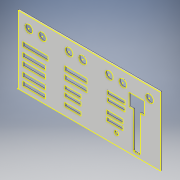
# Autodesk Inventor part: CNC - Tool Board
Saved by Autodesk Inventor 2017 SP1 (Build 210196100, 196)
## iProperties
Created: 2017-08-31
Part Number: CNC - Tool Board
Material: Generic
Document SubType Name: Modeling
Designer: rmainhar
Density: 1 g/cm^3
Appearance: Default
Author: rmainhar
Autodesk Inventor part; units mm, degrees
ref_plane "YZ Plane" through (0, 0, 0) normal (1, 0, 0) x (0, 1, 0)
ref_plane "XZ Plane" through (0, 0, 0) normal (0, 1, 0) x (-1, 0, 0)
ref_plane "XY Plane" through (0, 0, 0) normal (0, 0, 1) x (1, 0, 0)
sketch "Sketch1" plane through (0, 0, 0) normal (0, 0, 1) x (1, 0, 0)
  line L0 (0, 0) -> (584.2, 0)
  line L1 (584.2, 0) -> (584.2, 279.4)
  line L2 (584.2, 279.4) -> (0, 279.4)
  line L3 (0, 279.4) -> (0, 0)
  dimension "d0" = 584.2
  dimension "d1" = 279.4
  constraints: 8 end point, 2 parallel, 1 horizontal, 1 perpendicular
  measures "d0" distance of L2.end L1.end
  measures "d1" distance of L1.end L0.end
extrude "Extrusion1" add sketch "Sketch1" along normal blind 6.35
sketch "Sketch2" plane through (0, 0, 6.35) normal (0, 0, 1) x (1, 0, 0)
  circle A0 centre (43.6149, 234.95) radius 15.875
  circle A1 centre (99.4949, 234.95) radius 15.875
  line L0 (584.2, 279.4) -> (0, 279.4) projected
  circle A2 centre (208.7149, 234.95) radius 15.875
  circle A3 centre (264.5949, 234.95) radius 15.875
  circle A4 centre (373.8149, 234.95) radius 15.875
  circle A5 centre (429.6949, 234.95) radius 15.875
  circle A6 centre (538.9149, 234.95) radius 15.875
  circle A7 centre (594.7949, 234.95) radius 15.875
  point P0 (0, 0)
  dimension "d4" = 31.75
  dimension "d5" = 31.75
  dimension "d6" = 55.88
  dimension "d7" = 44.45
  dimension "d8" = 44.45
  dimension "d11" = 165.1
  constraints: 8 centre point, 1 horizontal, 12 other
  measures "d4" diameter of A0
  measures "d5" diameter of A1
  measures "d6" distance of A1.centre A0.centre
  measures "d7" distance from line of A1.centre L0
  measures "d8" distance from line of L0 A0.centre
  measures "d11" distance of A0.centre A2.centre
extrude "Extrusion2" cut sketch "Sketch2" against normal through all contours A0 | A1 | A2 | A3 | A4 | A5 | A6
sketch "Sketch3" plane through (0, 0, 6.35) normal (0, 0, 1) x (1, 0, 0)
  circle A0 centre (429.6949, 234.95) radius 15.875 projected
  circle A1 centre (264.5949, 234.95) radius 15.875 projected
  circle A2 centre (99.4949, 234.95) radius 15.875 projected
  circle A3 centre (43.6149, 234.95) radius 15.875 projected
  circle A4 centre (208.7149, 234.95) radius 15.875 projected
  circle A5 centre (373.8149, 234.95) radius 15.875 projected
  circle A6 centre (538.9149, 234.95) radius 15.875 projected
  line L0 (0, 0) -> (584.2, 0) projected
  line L1 (584.2, 0) -> (584.2, 279.4) projected
  line L2 (584.2, 279.4) -> (0, 279.4) projected
  line L3 (0, 279.4) -> (0, 0) projected
  line L4 (19.05, 177.8) -> (121.92, 177.8)
  line L5 (121.92, 177.8) -> (121.92, 158.75)
  line L6 (121.92, 158.75) -> (19.05, 158.75)
  line L7 (19.05, 158.75) -> (19.05, 177.8)
  line L8 (19.05, 139.7) -> (111.125, 139.7)
  line L9 (111.125, 139.7) -> (111.125, 120.65)
  line L10 (111.125, 120.65) -> (19.05, 120.65)
  line L11 (19.05, 120.65) -> (19.05, 139.7)
  line L12 (111.125, 107.95) -> (111.125, 88.9)
  line L13 (19.05, 107.95) -> (111.125, 107.95)
  line L14 (111.125, 88.9) -> (19.05, 88.9)
  line L15 (19.05, 88.9) -> (19.05, 107.95)
  line L16 (19.05, 50.8) -> (19.05, 69.85)
  line L17 (19.05, 19.05) -> (19.05, 38.1)
  line L18 (19.05, 69.85) -> (111.125, 69.85)
  line L19 (111.125, 69.85) -> (111.125, 50.8)
  line L20 (111.125, 50.8) -> (19.05, 50.8)
  line L21 (19.05, 38.1) -> (111.125, 38.1)
  line L22 (111.125, 38.1) -> (111.125, 19.05)
  line L23 (111.125, 19.05) -> (19.05, 19.05)
  dimension "d18" = 101.6
  dimension "d19" = 19.05
  dimension "d20" = 102.87
  dimension "d21" = 19.05
  dimension "d22" = 19.05
  dimension "d23" = 92.075
  dimension "d24" = 19.05
  dimension "d25" = 92.075
  dimension "d26" = 19.05
  dimension "d27" = 19.05
  dimension "d28" = 139.7
  dimension "d29" = 171.45
  dimension "d32" = 69.85
  constraints: 40 end point, 6 parallel, 3 horizontal, 3 perpendicular, 1 vertical, 16 other
  measures "d18" distance between parallel lines of L2 L4
  measures "d19" distance of L4.end L5.end
  measures "d20" distance between parallel lines of L5 L7
  measures "d21" distance between parallel lines of L3 L7
  measures "d22" distance of L9.start L9.end
  measures "d23" distance between parallel lines of L9 L11
  measures "d24" distance of L12.start L12.end
  measures "d25" distance between parallel lines of L12 L15
  measures "d26" distance between parallel lines of L3 L11
  measures "d27" distance between parallel lines of L15 L3
  measures "d28" distance between parallel lines of L2 L8
  measures "d29" distance between parallel lines of L2 L13
  measures "d32" distance of L8.start L16.end
extrude "Extrusion3" cut sketch "Sketch3" against normal through all contours L4 L5 L6 L7 | L8 L9 L10 L11 | L12 L14 L15 L13 | L16 L18 L19 L20 | L17 L21 L22 L23
sketch "Sketch4" plane through (0, 0, 6.35) normal (0, 0, 1) x (1, 0, 0)
  line L0 (19.05, 19.05) -> (19.05, 38.1) projected
  line L1 (19.05, 38.1) -> (111.125, 38.1) projected
  line L2 (111.125, 38.1) -> (111.125, 19.05) projected
  line L3 (111.125, 19.05) -> (19.05, 19.05) projected
  line L4 (19.05, 88.9) -> (19.05, 107.95) projected
  line L5 (19.05, 107.95) -> (111.125, 107.95) projected
  line L6 (111.125, 107.95) -> (111.125, 88.9) projected
  line L7 (111.125, 88.9) -> (19.05, 88.9) projected
  line L8 (19.05, 120.65) -> (19.05, 139.7) projected
  line L9 (19.05, 139.7) -> (111.125, 139.7) projected
  line L10 (111.125, 139.7) -> (111.125, 120.65) projected
  line L11 (111.125, 120.65) -> (19.05, 120.65) projected
  line L12 (19.05, 50.8) -> (19.05, 69.85) projected
  line L13 (19.05, 69.85) -> (111.125, 69.85) projected
  line L14 (111.125, 69.85) -> (111.125, 50.8) projected
  line L15 (111.125, 50.8) -> (19.05, 50.8) projected
  line L16 (19.05, 158.75) -> (19.05, 177.8) projected
  line L17 (19.05, 177.8) -> (121.92, 177.8) projected
  line L18 (121.92, 177.8) -> (121.92, 158.75) projected
  line L19 (121.92, 158.75) -> (19.05, 158.75) projected
  circle A0 centre (429.6949, 234.95) radius 15.875 projected
  circle A1 centre (264.5949, 234.95) radius 15.875 projected
  circle A2 centre (99.4949, 234.95) radius 15.875 projected
  circle A3 centre (43.6149, 234.95) radius 15.875 projected
  circle A4 centre (208.7149, 234.95) radius 15.875 projected
  circle A5 centre (373.8149, 234.95) radius 15.875 projected
  circle A6 centre (538.9149, 234.95) radius 15.875 projected
  line L20 (0, 0) -> (584.2, 0) projected
  line L21 (584.2, 0) -> (584.2, 279.4) projected
  line L22 (584.2, 279.4) -> (0, 279.4) projected
  line L23 (0, 279.4) -> (0, 0) projected
  line L24 (190.5, 158.75) -> (190.5, 177.8)
  line L25 (190.5, 177.8) -> (282.575, 177.8)
  line L26 (282.575, 177.8) -> (282.575, 158.75)
  line L27 (282.575, 158.75) -> (190.5, 158.75)
  line L28 (282.575, 146.05) -> (282.575, 127)
  line L29 (190.5, 127) -> (190.5, 146.05)
  line L30 (190.5, 146.05) -> (282.575, 146.05)
  line L31 (282.575, 127) -> (190.5, 127)
  line L32 (190.5, 107.95) -> (257.175, 107.95)
  line L33 (257.175, 107.95) -> (257.175, 92.075)
  line L34 (257.175, 92.075) -> (190.5, 92.075)
  line L35 (190.5, 92.075) -> (190.5, 107.95)
  line L36 (190.5, 82.55) -> (257.175, 82.55)
  line L37 (257.175, 82.55) -> (257.175, 66.675)
  line L38 (257.175, 66.675) -> (190.5, 66.675)
  line L39 (190.5, 66.675) -> (190.5, 82.55)
  line L40 (190.5, 47.625) -> (257.175, 47.625)
  line L41 (257.175, 47.625) -> (257.175, 31.75)
  line L42 (257.175, 31.75) -> (190.5, 31.75)
  line L43 (190.5, 31.75) -> (190.5, 47.625)
  dimension "d39" = 19.05
  dimension "d40" = 92.075
  dimension "d41" = 190.5
  dimension "d42" = 19.05
  dimension "d43" = 92.075
  dimension "d44" = 190.5
  dimension "d45" = 133.35
  dimension "d46" = 101.6
  dimension "d47" = 66.675
  dimension "d48" = 15.875
  dimension "d49" = 171.45
  dimension "d50" = 190.5
  dimension "d51" = 66.675
  dimension "d52" = 15.875
  dimension "d53" = 190.5
  dimension "d54" = 196.85
  dimension "d55" = 66.675
  dimension "d56" = 15.875
  dimension "d57" = 231.775
  dimension "d58" = 190.5
  constraints: 40 end point, 9 perpendicular, 6 parallel, 3 horizontal
  measures "d39" distance of L26.start L26.end
  measures "d40" distance of L24.end L26.start
  measures "d41" distance between parallel lines of L23 L24
  measures "d42" distance of L28.start L28.end
  measures "d43" distance of L29.end L28.start
  measures "d44" distance between parallel lines of L23 L29
  measures "d45" distance between parallel lines of L22 L30
  measures "d46" distance between parallel lines of L22 L25
  measures "d47" distance of L33.end L34.end
  measures "d48" distance of L32.end L33.end
  measures "d49" distance between parallel lines of L22 L32
  measures "d50" distance between parallel lines of L23 L35
  measures "d51" distance of L38.start L39.start
  measures "d52" distance of L36.end L38.start
  measures "d53" distance between parallel lines of L39 L23
  measures "d54" distance between parallel lines of L22 L36
  measures "d55" distance of L42.start L43.start
  measures "d56" distance of L40.end L42.start
  measures "d57" distance between parallel lines of L22 L40
  measures "d58" distance between parallel lines of L23 L43
extrude "Extrusion4" cut sketch "Sketch4" against normal through all contours L24 L25 L26 L27 | L28 L31 L29 L30 | L32 L33 L34 L35 | L36 L37 L38 L39 | L40 L41 L42 L43
sketch "Sketch5" plane through (0, 0, 6.35) normal (0, 0, 1) x (1, 0, 0)
  line L0 (190.5, 158.75) -> (190.5, 177.8) projected
  line L1 (190.5, 177.8) -> (282.575, 177.8) projected
  line L2 (282.575, 177.8) -> (282.575, 158.75) projected
  line L3 (282.575, 158.75) -> (190.5, 158.75) projected
  line L4 (190.5, 66.675) -> (190.5, 82.55) projected
  line L5 (190.5, 82.55) -> (257.175, 82.55) projected
  line L6 (257.175, 82.55) -> (257.175, 66.675) projected
  line L7 (257.175, 66.675) -> (190.5, 66.675) projected
  line L8 (190.5, 92.075) -> (190.5, 107.95) projected
  line L9 (190.5, 107.95) -> (257.175, 107.95) projected
  line L10 (257.175, 107.95) -> (257.175, 92.075) projected
  line L11 (257.175, 92.075) -> (190.5, 92.075) projected
  line L12 (190.5, 31.75) -> (190.5, 47.625) projected
  line L13 (190.5, 47.625) -> (257.175, 47.625) projected
  line L14 (257.175, 47.625) -> (257.175, 31.75) projected
  line L15 (257.175, 31.75) -> (190.5, 31.75) projected
  line L16 (282.575, 127) -> (190.5, 127) projected
  line L17 (190.5, 127) -> (190.5, 146.05) projected
  line L18 (190.5, 146.05) -> (282.575, 146.05) projected
  line L19 (282.575, 146.05) -> (282.575, 127) projected
  line L20 (19.05, 19.05) -> (19.05, 38.1) projected
  line L21 (19.05, 38.1) -> (111.125, 38.1) projected
  line L22 (111.125, 38.1) -> (111.125, 19.05) projected
  line L23 (111.125, 19.05) -> (19.05, 19.05) projected
  line L24 (19.05, 88.9) -> (19.05, 107.95) projected
  line L25 (19.05, 107.95) -> (111.125, 107.95) projected
  line L26 (111.125, 107.95) -> (111.125, 88.9) projected
  line L27 (111.125, 88.9) -> (19.05, 88.9) projected
  line L28 (19.05, 120.65) -> (19.05, 139.7) projected
  line L29 (19.05, 139.7) -> (111.125, 139.7) projected
  line L30 (111.125, 139.7) -> (111.125, 120.65) projected
  line L31 (111.125, 120.65) -> (19.05, 120.65) projected
  line L32 (19.05, 50.8) -> (19.05, 69.85) projected
  line L33 (19.05, 69.85) -> (111.125, 69.85) projected
  line L34 (111.125, 69.85) -> (111.125, 50.8) projected
  line L35 (111.125, 50.8) -> (19.05, 50.8) projected
  line L36 (19.05, 158.75) -> (19.05, 177.8) projected
  line L37 (19.05, 177.8) -> (121.92, 177.8) projected
  line L38 (121.92, 177.8) -> (121.92, 158.75) projected
  line L39 (121.92, 158.75) -> (19.05, 158.75) projected
  circle A0 centre (429.6949, 234.95) radius 15.875 projected
  circle A1 centre (264.5949, 234.95) radius 15.875 projected
  circle A2 centre (99.4949, 234.95) radius 15.875 projected
  circle A3 centre (43.6149, 234.95) radius 15.875 projected
  circle A4 centre (208.7149, 234.95) radius 15.875 projected
  circle A5 centre (373.8149, 234.95) radius 15.875 projected
  circle A6 centre (538.9149, 234.95) radius 15.875 projected
  line L40 (0, 0) -> (584.2, 0) projected
  line L41 (584.2, 0) -> (584.2, 279.4) projected
  line L42 (584.2, 279.4) -> (0, 279.4) projected
  line L43 (0, 279.4) -> (0, 0) projected
  line L44 (365.125, 161.925) -> (365.125, 177.8)
  line L45 (365.125, 177.8) -> (438.15, 177.8)
  line L46 (438.15, 177.8) -> (438.15, 161.925)
  line L47 (438.15, 161.925) -> (365.125, 161.925)
  line L48 (365.125, 152.4) -> (438.15, 152.4)
  line L49 (365.125, 136.525) -> (365.125, 152.4)
  line L50 (438.15, 136.525) -> (365.125, 136.525)
  line L51 (438.15, 152.4) -> (438.15, 136.525)
  dimension "d61" = 15.875
  dimension "d62" = 73.025
  dimension "d63" = 101.6
  dimension "d64" = 365.125
  dimension "d67" = 25.4
  constraints: 16 end point, 3 perpendicular, 1 vertical, 8 other
  measures "d61" distance of L46.start L47.start
  measures "d62" distance of L44.end L46.start
  measures "d63" distance between parallel lines of L42 L45
  measures "d64" distance between parallel lines of L43 L44
  measures "d67" distance of L44.end L48.start
extrude "Extrusion5" cut sketch "Sketch5" against normal through all contours L44 L45 L46 L47 | L48 L51 L50 L49
sketch "Sketch6" plane through (0, 0, 6.35) normal (0, 0, 1) x (1, 0, 0)
  circle A0 centre (403.225, 44.45) radius 8.5725
  line L0 (584.2, 0) -> (584.2, 279.4) projected
  line L1 (0, 0) -> (584.2, 0) projected
  line L2 (472.1918, 165.1) -> (500.7668, 165.1)
  line L3 (500.7668, 165.1) -> (500.7668, 19.05)
  line L4 (494.4168, 12.7) -> (478.5418, 12.7)
  line L5 (472.1918, 19.05) -> (472.1918, 165.1)
  arc A1 (472.1918, 19.05) -> (478.5418, 12.7) centre (478.5418, 19.05) ccw
  arc A2 (494.4168, 12.7) -> (500.7668, 19.05) centre (494.4168, 19.05) ccw
  line L6 (455.0468, 215.9) -> (517.9118, 215.9)
  line L7 (517.9118, 215.9) -> (517.9118, 163.2742)
  line L8 (517.9118, 163.2742) -> (455.0468, 163.2742)
  line L9 (455.0468, 163.2742) -> (455.0468, 215.9)
  point P0 (500.7668, 12.7)
  dimension "d74" = 17.145
  dimension "d75" = 180.975
  dimension "d76" = 44.45
  dimension "d77" = 28.575
  dimension "d78" = 152.4
  dimension "d79" = 6.35
  dimension "d80" = 12.7
  dimension "d81" = 17.145
  dimension "d82" = 17.145
  dimension "d83" = 50.8
  constraints: 16 end point, 4 parallel, 4 point on circle, 4 tangent, 3 centre point, 2 horizontal, 2 perpendicular, 2 point on line, 1 equal radius
  measures "d74" diameter of A0
  measures "d75" distance from line of L0 A0.centre
  measures "d76" distance from line of L1 A0.centre
  measures "d77" distance of L2.start L2.end
  measures "d78" distance of L2.end point (500.767, 12.7)
  measures "d79" radius of A1
  measures "d80" distance between parallel lines of L1 L4
  measures "d81" distance between parallel lines of L7 L3
  measures "d82" distance between parallel lines of L5 L9
  measures "d83" distance between parallel lines of L2 L6
extrude "Extrusion6" cut sketch "Sketch6" against normal through all
sketch "Sketch8" plane through (0, 0, 6.35) normal (0, 0, 1) x (1, 0, 0)
  circle A0 centre (403.225, 44.45) radius 8.5725 projected
  line L0 (455.0468, 163.2742) -> (455.0468, 215.9) projected
  line L1 (455.0468, 215.9) -> (517.9118, 215.9) projected
  line L2 (517.9118, 215.9) -> (517.9118, 163.2742) projected
  line L3 (517.9118, 163.2742) -> (500.7668, 163.2742) projected
  line L4 (500.7668, 163.2742) -> (500.7668, 19.05) projected
  arc A1 (494.4168, 12.7) -> (500.7668, 19.05) centre (494.4168, 19.05) ccw projected
  line L5 (494.4168, 12.7) -> (478.5418, 12.7) projected
  arc A2 (472.1918, 19.05) -> (478.5418, 12.7) centre (478.5418, 19.05) ccw projected
  line L6 (472.1918, 19.05) -> (472.1918, 163.2742) projected
  line L7 (472.1918, 163.2742) -> (455.0468, 163.2742) projected
  line L8 (438.15, 161.925) -> (365.125, 161.925) projected
  line L9 (365.125, 161.925) -> (365.125, 177.8) projected
  line L10 (365.125, 177.8) -> (438.15, 177.8) projected
  line L11 (438.15, 177.8) -> (438.15, 161.925) projected
  line L12 (438.15, 136.525) -> (365.125, 136.525) projected
  line L13 (365.125, 136.525) -> (365.125, 152.4) projected
  line L14 (365.125, 152.4) -> (438.15, 152.4) projected
  line L15 (438.15, 152.4) -> (438.15, 136.525) projected
  line L16 (190.5, 158.75) -> (190.5, 177.8) projected
  line L17 (190.5, 177.8) -> (282.575, 177.8) projected
  line L18 (282.575, 177.8) -> (282.575, 158.75) projected
  line L19 (282.575, 158.75) -> (190.5, 158.75) projected
  line L20 (190.5, 66.675) -> (190.5, 82.55) projected
  line L21 (190.5, 82.55) -> (257.175, 82.55) projected
  line L22 (257.175, 82.55) -> (257.175, 66.675) projected
  line L23 (257.175, 66.675) -> (190.5, 66.675) projected
  line L24 (190.5, 92.075) -> (190.5, 107.95) projected
  line L25 (190.5, 107.95) -> (257.175, 107.95) projected
  line L26 (257.175, 107.95) -> (257.175, 92.075) projected
  line L27 (257.175, 92.075) -> (190.5, 92.075) projected
  line L28 (190.5, 31.75) -> (190.5, 47.625) projected
  line L29 (190.5, 47.625) -> (257.175, 47.625) projected
  line L30 (257.175, 47.625) -> (257.175, 31.75) projected
  line L31 (257.175, 31.75) -> (190.5, 31.75) projected
  line L32 (282.575, 127) -> (190.5, 127) projected
  line L33 (190.5, 127) -> (190.5, 146.05) projected
  line L34 (190.5, 146.05) -> (282.575, 146.05) projected
  line L35 (282.575, 146.05) -> (282.575, 127) projected
  line L36 (19.05, 19.05) -> (19.05, 38.1) projected
  line L37 (19.05, 38.1) -> (111.125, 38.1) projected
  line L38 (111.125, 38.1) -> (111.125, 19.05) projected
  line L39 (111.125, 19.05) -> (19.05, 19.05) projected
  line L40 (19.05, 88.9) -> (19.05, 107.95) projected
  line L41 (19.05, 107.95) -> (111.125, 107.95) projected
  line L42 (111.125, 107.95) -> (111.125, 88.9) projected
  line L43 (111.125, 88.9) -> (19.05, 88.9) projected
  line L44 (19.05, 120.65) -> (19.05, 139.7) projected
  line L45 (19.05, 139.7) -> (111.125, 139.7) projected
  line L46 (111.125, 139.7) -> (111.125, 120.65) projected
  line L47 (111.125, 120.65) -> (19.05, 120.65) projected
  line L48 (19.05, 50.8) -> (19.05, 69.85) projected
  line L49 (19.05, 69.85) -> (111.125, 69.85) projected
  line L50 (111.125, 69.85) -> (111.125, 50.8) projected
  line L51 (111.125, 50.8) -> (19.05, 50.8) projected
  line L52 (19.05, 158.75) -> (19.05, 177.8) projected
  line L53 (19.05, 177.8) -> (121.92, 177.8) projected
  line L54 (121.92, 177.8) -> (121.92, 158.75) projected
  line L55 (121.92, 158.75) -> (19.05, 158.75) projected
  circle A3 centre (429.6949, 234.95) radius 15.875 projected
  circle A4 centre (264.5949, 234.95) radius 15.875 projected
  circle A5 centre (99.4949, 234.95) radius 15.875 projected
  circle A6 centre (43.6149, 234.95) radius 15.875 projected
  circle A7 centre (208.7149, 234.95) radius 15.875 projected
  circle A8 centre (373.8149, 234.95) radius 15.875 projected
  circle A9 centre (538.9149, 234.95) radius 15.875 projected
  line L56 (0, 0) -> (584.2, 0) projected
  line L57 (584.2, 0) -> (584.2, 279.4) projected
  line L58 (584.2, 279.4) -> (0, 279.4) projected
  line L59 (0, 279.4) -> (0, 0) projected
  line L60 (362.9822, 107.3165) -> (429.6572, 107.3165)
  line L61 (429.6572, 107.3165) -> (429.6572, 90.6271)
  line L62 (429.6572, 90.6271) -> (362.9822, 90.6271)
  line L63 (362.9822, 90.6271) -> (362.9822, 107.3165)
  line L64 (362.9822, 82.0655) -> (429.6572, 82.0655)
  line L65 (429.6572, 82.0655) -> (429.6572, 66.2837)
  line L66 (429.6572, 66.2837) -> (362.9822, 66.2837)
  line L67 (362.9822, 66.2837) -> (362.9822, 82.0655)
  dimension "d86" = 66.675
  dimension "d87" = 66.675
  constraints: 16 end point, 4 parallel, 2 horizontal, 2 perpendicular
  measures "d86" distance of L60.start L60.end
  measures "d87" distance of L64.start L64.end
extrude "Extrusion7" cut sketch "Sketch8" against normal blind 6.35 contours L60 L61 L62 L63 | L64 L65 L66 L67
sketch "Sketch9" plane through (0, 0, 6.35) normal (0, 0, 1) x (1, 0, 0)
  line L0 (362.9822, 66.2837) -> (362.9822, 82.0655) projected
  line L1 (362.9822, 82.0655) -> (429.6572, 82.0655) projected
  line L2 (429.6572, 82.0655) -> (429.6572, 66.2837) projected
  line L3 (429.6572, 66.2837) -> (362.9822, 66.2837) projected
  line L4 (362.9822, 90.6271) -> (362.9822, 107.3165) projected
  line L5 (362.9822, 107.3165) -> (429.6572, 107.3165) projected
  line L6 (429.6572, 107.3165) -> (429.6572, 90.6271) projected
  line L7 (429.6572, 90.6271) -> (362.9822, 90.6271) projected
  circle A0 centre (403.225, 44.45) radius 8.5725 projected
  line L8 (455.0468, 163.2742) -> (455.0468, 215.9) projected
  line L9 (455.0468, 215.9) -> (517.9118, 215.9) projected
  line L10 (517.9118, 215.9) -> (517.9118, 163.2742) projected
  line L11 (517.9118, 163.2742) -> (500.7668, 163.2742) projected
  line L12 (500.7668, 163.2742) -> (500.7668, 19.05) projected
  arc A1 (494.4168, 12.7) -> (500.7668, 19.05) centre (494.4168, 19.05) ccw projected
  line L13 (494.4168, 12.7) -> (478.5418, 12.7) projected
  arc A2 (472.1918, 19.05) -> (478.5418, 12.7) centre (478.5418, 19.05) ccw projected
  line L14 (472.1918, 19.05) -> (472.1918, 163.2742) projected
  line L15 (472.1918, 163.2742) -> (455.0468, 163.2742) projected
  line L16 (438.15, 161.925) -> (365.125, 161.925) projected
  line L17 (365.125, 161.925) -> (365.125, 177.8) projected
  line L18 (365.125, 177.8) -> (438.15, 177.8) projected
  line L19 (438.15, 177.8) -> (438.15, 161.925) projected
  line L20 (438.15, 136.525) -> (365.125, 136.525) projected
  line L21 (365.125, 136.525) -> (365.125, 152.4) projected
  line L22 (365.125, 152.4) -> (438.15, 152.4) projected
  line L23 (438.15, 152.4) -> (438.15, 136.525) projected
  line L24 (190.5, 158.75) -> (190.5, 177.8) projected
  line L25 (190.5, 177.8) -> (282.575, 177.8) projected
  line L26 (282.575, 177.8) -> (282.575, 158.75) projected
  line L27 (282.575, 158.75) -> (190.5, 158.75) projected
  line L28 (190.5, 66.675) -> (190.5, 82.55) projected
  line L29 (190.5, 82.55) -> (257.175, 82.55) projected
  line L30 (257.175, 82.55) -> (257.175, 66.675) projected
  line L31 (257.175, 66.675) -> (190.5, 66.675) projected
  line L32 (190.5, 92.075) -> (190.5, 107.95) projected
  line L33 (190.5, 107.95) -> (257.175, 107.95) projected
  line L34 (257.175, 107.95) -> (257.175, 92.075) projected
  line L35 (257.175, 92.075) -> (190.5, 92.075) projected
  line L36 (190.5, 31.75) -> (190.5, 47.625) projected
  line L37 (190.5, 47.625) -> (257.175, 47.625) projected
  line L38 (257.175, 47.625) -> (257.175, 31.75) projected
  line L39 (257.175, 31.75) -> (190.5, 31.75) projected
  line L40 (282.575, 127) -> (190.5, 127) projected
  line L41 (190.5, 127) -> (190.5, 146.05) projected
  line L42 (190.5, 146.05) -> (282.575, 146.05) projected
  line L43 (282.575, 146.05) -> (282.575, 127) projected
  line L44 (19.05, 19.05) -> (19.05, 38.1) projected
  line L45 (19.05, 38.1) -> (111.125, 38.1) projected
  line L46 (111.125, 38.1) -> (111.125, 19.05) projected
  line L47 (111.125, 19.05) -> (19.05, 19.05) projected
  line L48 (19.05, 88.9) -> (19.05, 107.95) projected
  line L49 (19.05, 107.95) -> (111.125, 107.95) projected
  line L50 (111.125, 107.95) -> (111.125, 88.9) projected
  line L51 (111.125, 88.9) -> (19.05, 88.9) projected
  line L52 (19.05, 120.65) -> (19.05, 139.7) projected
  line L53 (19.05, 139.7) -> (111.125, 139.7) projected
  line L54 (111.125, 139.7) -> (111.125, 120.65) projected
  line L55 (111.125, 120.65) -> (19.05, 120.65) projected
  line L56 (19.05, 50.8) -> (19.05, 69.85) projected
  line L57 (19.05, 69.85) -> (111.125, 69.85) projected
  line L58 (111.125, 69.85) -> (111.125, 50.8) projected
  line L59 (111.125, 50.8) -> (19.05, 50.8) projected
  line L60 (19.05, 158.75) -> (19.05, 177.8) projected
  line L61 (19.05, 177.8) -> (121.92, 177.8) projected
  line L62 (121.92, 177.8) -> (121.92, 158.75) projected
  line L63 (121.92, 158.75) -> (19.05, 158.75) projected
  circle A3 centre (429.6949, 234.95) radius 15.875 projected
  circle A4 centre (264.5949, 234.95) radius 15.875 projected
  circle A5 centre (99.4949, 234.95) radius 15.875 projected
  circle A6 centre (43.6149, 234.95) radius 15.875 projected
  circle A7 centre (208.7149, 234.95) radius 15.875 projected
  circle A8 centre (373.8149, 234.95) radius 15.875 projected
  circle A9 centre (538.9149, 234.95) radius 15.875 projected
  line L64 (0, 0) -> (584.2, 0) projected
  line L65 (584.2, 0) -> (584.2, 279.4) projected
  line L66 (584.2, 279.4) -> (0, 279.4) projected
  line L67 (0, 279.4) -> (0, 0) projected
equation "\"d5\" = d4"
equation "\"d8\" = d7"
equation "\"d26\" = d21"
equation "\"d27\" = d26"
equation "\"d44\" = d41"
equation "\"d50\" = d41"
equation "\"d53\" = d41"
equation "\"d58\" = d41"
body "Solid1"
